Autodesk Fusion 360 part; units mm, degrees
(part 3 of 3)
sketch "Sketch8" plane through (0, 0, 8.15) normal (0, 0, 1) x (1, 0, 0) in component "Top"
extrude "Extrude4'" cut sketch "eaeb931b339a04fc4a439f0e48c97f53086cf32d_switch" along normal up to surface (1.5 mm away) contours L200 L201 L202 L203 bodies 1 in component "Plate"
sketch "Sketch9" plane through (0, 0, 8.15) normal (0, 0, 1) x (-1, 0, 0) in component "Top"
  line L0 (-81.77, -114.5353) -> (-67.7693, -114.5353)
  line L1 (-67.7693, -114.5353) -> (-67.7693, -128.5347)
  line L2 (-67.7693, -128.5347) -> (-81.77, -128.5347)
  line L3 (-81.77, -128.5347) -> (-81.77, -114.5353)
  circle A0 centre (-85.4771, -7.1284) radius 1
  circle A1 centre (-6.9121, -7.1284) radius 1
  circle A2 centre (-84.7093, -138.9743) radius 1
  line L4 (-81.77, -72.4598) -> (-81.77, -58.4606)
  line L5 (-81.77, -58.4606) -> (-77.0696, -58.4606)
  line L6 (-77.0696, -58.4606) -> (-77.0696, -56.9352)
  line L7 (-77.0696, -56.9352) -> (-80.2996, -56.9352)
  line L8 (-80.2996, -56.9352) -> (-80.2996, -55.2097)
  line L9 (-80.2996, -55.2097) -> (-81.219, -55.2097)
  line L10 (-81.219, -55.2097) -> (-81.219, -51.9105)
  line L11 (-81.219, -51.9105) -> (-80.2996, -51.9105)
  line L12 (-80.2996, -51.9105) -> (-80.2996, -50.1855)
  line L13 (-80.2996, -50.1855) -> (-77.0696, -50.1855)
  line L14 (-77.0696, -50.1855) -> (-77.0696, -49.36)
  line L15 (-77.0696, -49.36) -> (-74.2692, -49.36)
  line L16 (-74.2692, -49.36) -> (-74.2692, -50.1855)
  line L17 (-74.2692, -50.1855) -> (-67.9993, -50.1855)
  line L18 (-67.9993, -50.1855) -> (-67.9993, -51.9105)
  line L19 (-67.9993, -51.9105) -> (-67.0197, -51.9105)
  line L20 (-67.0197, -51.9105) -> (-67.0197, -55.2097)
  line L21 (-67.0197, -55.2097) -> (-67.9993, -55.2097)
  line L22 (-67.9993, -55.2097) -> (-67.9993, -56.9352)
  line L23 (-67.9993, -56.9352) -> (-72.4697, -56.9352)
  line L24 (-72.4697, -56.9352) -> (-72.4697, -58.4606)
  line L25 (-72.4697, -58.4606) -> (-67.7693, -58.4606)
  line L26 (-67.7693, -58.4606) -> (-67.7693, -72.4598)
  line L27 (-67.7693, -72.4598) -> (-72.4697, -72.4598)
  line L28 (-72.4697, -72.4598) -> (-72.4697, -73.9856)
  line L29 (-72.4697, -73.9856) -> (-67.9993, -73.9856)
  line L30 (-67.9993, -73.9856) -> (-67.9993, -75.7107)
  line L31 (-67.9993, -75.7107) -> (-67.0197, -75.7107)
  line L32 (-67.0197, -75.7107) -> (-67.0197, -79.0099)
  line L33 (-67.0197, -79.0099) -> (-67.9993, -79.0099)
  line L34 (-67.9993, -79.0099) -> (-67.9993, -80.735)
  line L35 (-67.9993, -80.735) -> (-74.2692, -80.735)
  line L36 (-74.2692, -80.735) -> (-74.2692, -81.5605)
  line L37 (-74.2692, -81.5605) -> (-77.0696, -81.5605)
  line L38 (-77.0696, -81.5605) -> (-77.0696, -80.735)
  line L39 (-77.0696, -80.735) -> (-80.2996, -80.735)
  line L40 (-80.2996, -80.735) -> (-80.2996, -79.0099)
  line L41 (-80.2996, -79.0099) -> (-81.219, -79.0099)
  line L42 (-81.219, -79.0099) -> (-81.219, -75.7107)
  line L43 (-81.219, -75.7107) -> (-80.2996, -75.7107)
  line L44 (-80.2996, -75.7107) -> (-80.2996, -73.9856)
  line L45 (-80.2996, -73.9856) -> (-77.0696, -73.9856)
  line L46 (-77.0696, -73.9856) -> (-77.0696, -72.4598)
  line L47 (-77.0696, -72.4598) -> (-81.77, -72.4598)
  line L48 (-24.62, -101.035) -> (-24.62, -87.0356)
  line L49 (-24.62, -87.0356) -> (-10.6192, -87.0356)
  line L50 (-10.6192, -87.0356) -> (-10.6192, -101.035)
  line L51 (-10.6192, -101.035) -> (-24.62, -101.035)
  line L52 (-31.4446, -129.035) -> (-60.9446, -129.035)
  line L53 (-60.9446, -129.035) -> (-60.9446, -114.035)
  line L54 (-60.9446, -114.035) -> (-31.4446, -114.035)
  line L55 (-31.4446, -114.035) -> (-31.4446, -129.035)
  line L56 (-10.6192, -114.5353) -> (-10.6192, -128.5347)
  line L57 (-10.6192, -128.5347) -> (-24.62, -128.5347)
  line L58 (-24.62, -128.5347) -> (-24.62, -114.5353)
  line L59 (-24.62, -114.5353) -> (-10.6192, -114.5353)
  line L60 (-24.62, -67.9856) -> (-10.6192, -67.9856)
  line L61 (-10.6192, -67.9856) -> (-10.6192, -81.9848)
  line L62 (-10.6192, -81.9848) -> (-24.62, -81.9848)
  line L63 (-24.62, -81.9848) -> (-24.62, -67.9856)
  line L64 (-48.7193, -101.035) -> (-62.72, -101.035)
  line L65 (-62.72, -101.035) -> (-62.72, -87.0356)
  line L66 (-62.72, -87.0356) -> (-48.7193, -87.0356)
  line L67 (-48.7193, -87.0356) -> (-48.7193, -101.035)
  line L68 (-81.77, -87.0356) -> (-67.7693, -87.0356)
  line L69 (-67.7693, -87.0356) -> (-67.7693, -101.035)
  line L70 (-67.7693, -101.035) -> (-81.77, -101.035)
  line L71 (-81.77, -101.035) -> (-81.77, -87.0356)
  line L72 (-62.72, -67.9856) -> (-48.7193, -67.9856)
  line L73 (-48.7193, -67.9856) -> (-48.7193, -81.9848)
  line L74 (-48.7193, -81.9848) -> (-62.72, -81.9848)
  line L75 (-62.72, -81.9848) -> (-62.72, -67.9856)
  line L76 (-29.6692, -67.9856) -> (-29.6692, -81.9848)
  line L77 (-29.6692, -81.9848) -> (-43.67, -81.9848)
  line L78 (-43.67, -81.9848) -> (-43.67, -67.9856)
  line L79 (-43.67, -67.9856) -> (-29.6692, -67.9856)
  line L80 (-29.6692, -48.9356) -> (-29.6692, -62.9348)
  line L81 (-29.6692, -62.9348) -> (-43.67, -62.9348)
  line L82 (-43.67, -62.9348) -> (-43.67, -48.9356)
  line L83 (-43.67, -48.9356) -> (-29.6692, -48.9356)
  line L84 (-67.9993, -12.0854) -> (-67.9993, -13.8107)
  line L85 (-67.9993, -13.8107) -> (-67.0197, -13.8107)
  line L86 (-67.0197, -13.8107) -> (-67.0197, -17.1097)
  line L87 (-67.0197, -17.1097) -> (-67.9993, -17.1097)
  line L88 (-67.9993, -17.1097) -> (-67.9993, -18.835)
  line L89 (-67.9993, -18.835) -> (-72.4697, -18.835)
  line L90 (-72.4697, -18.835) -> (-72.4697, -20.3605)
  line L91 (-72.4697, -20.3605) -> (-67.7693, -20.3605)
  line L92 (-67.7693, -20.3605) -> (-67.7693, -34.36)
  line L93 (-67.7693, -34.36) -> (-72.4697, -34.36)
  line L94 (-72.4697, -34.36) -> (-72.4697, -35.8856)
  line L95 (-72.4697, -35.8856) -> (-67.9993, -35.8856)
  line L96 (-67.9993, -35.8856) -> (-67.9993, -37.6107)
  line L97 (-67.9993, -37.6107) -> (-67.0197, -37.6107)
  line L98 (-67.0197, -37.6107) -> (-67.0197, -40.9099)
  line L99 (-67.0197, -40.9099) -> (-67.9993, -40.9099)
  line L100 (-67.9993, -40.9099) -> (-67.9993, -42.635)
  line L101 (-67.9993, -42.635) -> (-74.2692, -42.635)
  line L102 (-74.2692, -42.635) -> (-74.2692, -43.4605)
  line L103 (-74.2692, -43.4605) -> (-77.0696, -43.4605)
  line L104 (-77.0696, -43.4605) -> (-77.0696, -42.635)
  line L105 (-77.0696, -42.635) -> (-80.2996, -42.635)
  line L106 (-80.2996, -42.635) -> (-80.2996, -40.9099)
  line L107 (-80.2996, -40.9099) -> (-81.219, -40.9099)
  line L108 (-81.219, -40.9099) -> (-81.219, -37.6107)
  line L109 (-81.219, -37.6107) -> (-80.2996, -37.6107)
  line L110 (-80.2996, -37.6107) -> (-80.2996, -35.8856)
  line L111 (-80.2996, -35.8856) -> (-77.0696, -35.8856)
  line L112 (-77.0696, -35.8856) -> (-77.0696, -34.36)
  line L113 (-77.0696, -34.36) -> (-81.77, -34.36)
  line L114 (-81.77, -34.36) -> (-81.77, -20.3605)
  line L115 (-81.77, -20.3605) -> (-77.0696, -20.3605)
  line L116 (-77.0696, -20.3605) -> (-77.0696, -18.835)
  line L117 (-77.0696, -18.835) -> (-80.2996, -18.835)
  line L118 (-80.2996, -18.835) -> (-80.2996, -17.1097)
  line L119 (-80.2996, -17.1097) -> (-81.219, -17.1097)
  line L120 (-81.219, -17.1097) -> (-81.219, -13.8107)
  line L121 (-81.219, -13.8107) -> (-80.2996, -13.8107)
  line L122 (-80.2996, -13.8107) -> (-80.2996, -12.0854)
  line L123 (-80.2996, -12.0854) -> (-77.0696, -12.0854)
  line L124 (-77.0696, -12.0854) -> (-77.0696, -11.26)
  line L125 (-77.0696, -11.26) -> (-74.2692, -11.26)
  line L126 (-74.2692, -11.26) -> (-74.2692, -12.0854)
  line L127 (-74.2692, -12.0854) -> (-67.9993, -12.0854)
  line L128 (-48.7193, -62.9348) -> (-62.72, -62.9348)
  line L129 (-62.72, -62.9348) -> (-62.72, -48.9356)
  line L130 (-62.72, -48.9356) -> (-48.7193, -48.9356)
  line L131 (-48.7193, -48.9356) -> (-48.7193, -62.9348)
  line L132 (-48.7193, -10.8355) -> (-48.7193, -24.835)
  line L133 (-48.7193, -24.835) -> (-62.72, -24.835)
  line L134 (-62.72, -24.835) -> (-62.72, -10.8355)
  line L135 (-62.72, -10.8355) -> (-48.7193, -10.8355)
  line L136 (-37.3944, -23.3646) -> (-37.3944, -24.2852)
  line L137 (-37.3944, -24.2852) -> (-40.6936, -24.2852)
  line L138 (-40.6936, -24.2852) -> (-40.6936, -23.3646)
  line L139 (-40.6936, -23.3646) -> (-42.4187, -23.3646)
  line L140 (-42.4187, -23.3646) -> (-42.4187, -20.1345)
  line L141 (-42.4187, -20.1345) -> (-43.2442, -20.1345)
  line L142 (-43.2442, -20.1345) -> (-43.2442, -17.3357)
  line L143 (-43.2442, -17.3357) -> (-42.4187, -17.3357)
  line L144 (-42.4187, -17.3357) -> (-42.4187, -11.0657)
  line L145 (-42.4187, -11.0657) -> (-40.6936, -11.0657)
  line L146 (-40.6936, -11.0657) -> (-40.6936, -10.0858)
  line L147 (-40.6936, -10.0858) -> (-37.3944, -10.0858)
  line L148 (-37.3944, -10.0858) -> (-37.3944, -11.0657)
  line L149 (-37.3944, -11.0657) -> (-35.669, -11.0657)
  line L150 (-35.669, -11.0657) -> (-35.669, -15.5346)
  line L151 (-35.669, -15.5346) -> (-34.145, -15.5346)
  line L152 (-34.145, -15.5346) -> (-34.145, -10.8355)
  line L153 (-34.145, -10.8355) -> (-20.1442, -10.8355)
  line L154 (-20.1442, -10.8355) -> (-20.1442, -15.5346)
  line L155 (-20.1442, -15.5346) -> (-18.6201, -15.5346)
  line L156 (-18.6201, -15.5346) -> (-18.6201, -11.0657)
  line L157 (-18.6201, -11.0657) -> (-16.8934, -11.0657)
  line L158 (-16.8934, -11.0657) -> (-16.8934, -10.0858)
  line L159 (-16.8934, -10.0858) -> (-13.593, -10.0858)
  line L160 (-13.593, -10.0858) -> (-13.593, -11.0657)
  line L161 (-13.593, -11.0657) -> (-11.869, -11.0657)
  line L162 (-11.869, -11.0657) -> (-11.869, -17.3357)
  line L163 (-11.869, -17.3357) -> (-11.0436, -17.3357)
  line L164 (-11.0436, -17.3357) -> (-11.0436, -20.1345)
  line L165 (-11.0436, -20.1345) -> (-11.869, -20.1345)
  line L166 (-11.869, -20.1345) -> (-11.869, -23.3646)
  line L167 (-11.869, -23.3646) -> (-13.593, -23.3646)
  line L168 (-13.593, -23.3646) -> (-13.593, -24.2852)
  line L169 (-13.593, -24.2852) -> (-16.8934, -24.2852)
  line L170 (-16.8934, -24.2852) -> (-16.8934, -23.3646)
  line L171 (-16.8934, -23.3646) -> (-18.6201, -23.3646)
  line L172 (-18.6201, -23.3646) -> (-18.6201, -20.1345)
  line L173 (-18.6201, -20.1345) -> (-20.1442, -20.1345)
  line L174 (-20.1442, -20.1345) -> (-20.1442, -24.835)
  line L175 (-20.1442, -24.835) -> (-34.145, -24.835)
  line L176 (-34.145, -24.835) -> (-34.145, -20.1345)
  line L177 (-34.145, -20.1345) -> (-35.669, -20.1345)
  line L178 (-35.669, -20.1345) -> (-35.669, -23.3646)
  line L179 (-35.669, -23.3646) -> (-37.3944, -23.3646)
  line L180 (-62.72, -43.8849) -> (-62.72, -29.8855)
  line L181 (-62.72, -29.8855) -> (-48.7193, -29.8855)
  line L182 (-48.7193, -29.8855) -> (-48.7193, -43.8849)
  line L183 (-48.7193, -43.8849) -> (-62.72, -43.8849)
  line L184 (-24.62, -62.9348) -> (-24.62, -48.9356)
  line L185 (-24.62, -48.9356) -> (-10.6192, -48.9356)
  line L186 (-10.6192, -48.9356) -> (-10.6192, -62.9348)
  line L187 (-10.6192, -62.9348) -> (-24.62, -62.9348)
  line L188 (-43.67, -87.0356) -> (-29.6692, -87.0356)
  line L189 (-29.6692, -87.0356) -> (-29.6692, -101.035)
  line L190 (-29.6692, -101.035) -> (-43.67, -101.035)
  line L191 (-43.67, -101.035) -> (-43.67, -87.0356)
  line L192 (-24.62, -43.8849) -> (-24.62, -29.8855)
  line L193 (-24.62, -29.8855) -> (-10.6192, -29.8855)
  line L194 (-10.6192, -29.8855) -> (-10.6192, -43.8849)
  line L195 (-10.6192, -43.8849) -> (-24.62, -43.8849)
  line L196 (-29.6692, -29.8855) -> (-29.6692, -43.8849)
  line L197 (-29.6692, -43.8849) -> (-43.67, -43.8849)
  line L198 (-43.67, -43.8849) -> (-43.67, -29.8855)
  line L199 (-43.67, -29.8855) -> (-29.6692, -29.8855)
  arc A3 (-6.6192, -142.035) -> (-4.6192, -140.035) centre (-6.6192, -140.035) ccw
  line L200 (-4.6192, -140.035) -> (-4.6192, -6.8355)
  arc A4 (-4.6192, -6.8355) -> (-6.6192, -4.8355) centre (-6.6192, -6.8355) ccw
  line L201 (-6.6192, -4.8355) -> (-85.77, -4.8355)
  arc A5 (-85.77, -4.8355) -> (-87.77, -6.8355) centre (-85.77, -6.8355) ccw
  line L202 (-87.77, -6.8355) -> (-87.77, -140.035)
  arc A6 (-87.77, -140.035) -> (-85.77, -142.035) centre (-85.77, -140.035) ccw
  line L203 (-85.77, -142.035) -> (-6.6192, -142.035)
extrude "Extrude11" cut sketch "Sketch9" against normal up to surface (6.65 mm away) contours L52 L53 L54 L55 bodies 2 in component "Top"
fillet "Fillet6" radius 1 4 edges at (60.9446, 129.035, 4.9) (31.4446, 129.035, 4.9) (31.4446, 114.035, 4.9) (60.9446, 114.035, 4.9) on bodies 2 in component "Top"
extrude "Extrude10" [suppressed] in component "Top"
ref_plane "WorkPlane3" through (46.1946, 67.8413, 1.075) normal (0, 0, -1) x (-1, 0, 0) in component "Top"
sketch "Sketch2 (2)" plane through (0, 0, -13) normal (0, 0, -1) x (1, 0, 0) in component "Bottom"
  arc A0 (-1.5308, 3.3145) -> (-3.5308, 1.3145) centre (-1.5308, 1.3145) ccw
  line L0 (-3.5308, 1.3145) -> (-3.5308, -136.997)
  arc A1 (-3.5308, -136.997) -> (-1.5308, -138.997) centre (-1.5308, -136.997) ccw
  line L1 (-1.5308, -138.997) -> (93.92, -138.997)
  arc A2 (93.92, -138.997) -> (95.92, -136.997) centre (93.92, -136.997) ccw
  line L2 (95.92, -136.997) -> (95.92, 1.3145)
  arc A3 (95.92, 1.3145) -> (93.92, 3.3145) centre (93.92, 1.3145) ccw
  line L3 (93.92, 3.3145) -> (-1.5308, 3.3145)
  line L4 (-3.5308, -138.997) -> (0.4692, -138.997) construction
  line L5 (0.4692, -138.997) -> (0.4692, -134.997) construction
  line L6 (0.4692, -134.997) -> (-3.5308, -134.997) construction
  line L7 (-3.5308, -138.997) -> (-3.5308, -134.997) construction
  circle A4 centre (0.4692, -134.997) radius 1.5
  dimension "d137" = 4
  dimension "d138" = 4
  dimension "d139" = 3
  constraint perpendicular L0 L4
  constraint perpendicular L4 L5
  constraint coincident L0 L6.end
  constraint perpendicular L0 L6
  constraint perpendicular L6 L7
  constraint coincident L5.end L6.start
  measures "d137" distance of L4.start L4.end
  measures "d138" distance of L4.end L5.end
  measures "d139" diameter of A4
extrude "Extrude8" [suppressed] in component "Top"
extrude "Extrude2''" [no effect] in component "Lit Stripe"
extrude "Extrude2'''" [no effect] in component "Bottom"
mirror "Mirror3" [suppressed] in component "Top"
mirror "Mirror1''" [no effect] in component "Lit Stripe"
mirror "Mirror1'''" [no effect] in component "Bottom"
mirror "Mirror4" [suppressed] in component "Top"
mirror "Mirror2''" [no effect] in component "Lit Stripe"
mirror "Mirror2'''" [no effect] in component "Bottom"
sketch "Sketch3 (3)" plane through (0, 0, -13) normal (0, 0, -1) x (1, 0, 0) in component "Bottom"
  circle A0 centre (91.92, -0.6855) radius 1.5
  circle A1 centre (0.4692, -0.6855) radius 1.5
  circle A2 centre (91.92, -134.997) radius 1.5
  circle A3 centre (0.4692, -134.997) radius 1.5
  arc A4 (-1.5308, 3.3145) -> (-3.5308, 1.3145) centre (-1.5308, 1.3145) ccw
  line L0 (-3.5308, 1.3145) -> (-3.5308, -136.997)
  arc A5 (-3.5308, -136.997) -> (-1.5308, -138.997) centre (-1.5308, -136.997) ccw
  line L1 (-1.5308, -138.997) -> (93.92, -138.997)
  arc A6 (93.92, -138.997) -> (95.92, -136.997) centre (93.92, -136.997) ccw
  line L2 (95.92, -136.997) -> (95.92, 1.3145)
  arc A7 (95.92, 1.3145) -> (93.92, 3.3145) centre (93.92, 1.3145) ccw
  line L3 (93.92, 3.3145) -> (-1.5308, 3.3145)
  line L4 (91.92, -0.6855) -> (91.92, -134.997) construction
  line L5 (95.92, -67.8413) -> (-3.5308, -67.8412) construction
  circle A8 centre (91.92, -67.8413) radius 1.5
  dimension "d152" = 3
  constraint coincident A0.centre L4.start
  constraint coincident A2.centre L4.end
  constraint midpoint L2 L5.start
  constraint midpoint L0 L5.end
  constraint midpoint L4 A8.centre
  measures "d152" diameter of A8
extrude "Extrude9" [suppressed] in component "Top"
extrude "Extrude3''" [no effect] in component "Lit Stripe"
extrude "Extrude3'''" [no effect] in component "Bottom"
mirror "Mirror5" [suppressed] in component "Top"
mirror "Mirror3'" [no effect] in component "Lit Stripe"
mirror "Mirror3''" [no effect] in component "Bottom"
sketch "Sketch4 (2)" plane through (0, 0, 1.5) normal (0, 0, 1) x (-1, 0, 0) in component "Top"
  circle A0 centre (-85.4771, -7.1284) radius 1
  circle A1 centre (-6.9121, -7.1284) radius 1
  circle A2 centre (-84.4771, -127.5541) radius 1
  circle A3 centre (-7.9121, -127.5541) radius 1
  line L0 (-34.1946, -124.3473) -> (-58.1946, -124.3473)
  line L1 (-58.1946, -124.3473) -> (-58.1946, -111.3473)
  line L2 (-58.1946, -111.3473) -> (-34.1946, -111.3473)
  line L3 (-34.1946, -111.3473) -> (-34.1946, -124.3473)
  line L4 (-81.77, -72.4598) -> (-81.77, -58.4606)
  line L5 (-81.77, -58.4606) -> (-77.0696, -58.4606)
  line L6 (-77.0696, -58.4606) -> (-77.0696, -56.9352)
  line L7 (-77.0696, -56.9352) -> (-80.2996, -56.9352)
  line L8 (-80.2996, -56.9352) -> (-80.2996, -55.2097)
  line L9 (-80.2996, -55.2097) -> (-81.219, -55.2097)
  line L10 (-81.219, -55.2097) -> (-81.219, -51.9105)
  line L11 (-81.219, -51.9105) -> (-80.2996, -51.9105)
  line L12 (-80.2996, -51.9105) -> (-80.2996, -50.1855)
  line L13 (-80.2996, -50.1855) -> (-77.0696, -50.1855)
  line L14 (-77.0696, -50.1855) -> (-77.0696, -49.36)
  line L15 (-77.0696, -49.36) -> (-74.2692, -49.36)
  line L16 (-74.2692, -49.36) -> (-74.2692, -50.1855)
  line L17 (-74.2692, -50.1855) -> (-67.9993, -50.1855)
  line L18 (-67.9993, -50.1855) -> (-67.9993, -51.9105)
  line L19 (-67.9993, -51.9105) -> (-67.0197, -51.9105)
  line L20 (-67.0197, -51.9105) -> (-67.0197, -55.2097)
  line L21 (-67.0197, -55.2097) -> (-67.9993, -55.2097)
  line L22 (-67.9993, -55.2097) -> (-67.9993, -56.9352)
  line L23 (-67.9993, -56.9352) -> (-72.4697, -56.9352)
  line L24 (-72.4697, -56.9352) -> (-72.4697, -58.4606)
  line L25 (-72.4697, -58.4606) -> (-67.7693, -58.4606)
  line L26 (-67.7693, -58.4606) -> (-67.7693, -72.4598)
  line L27 (-67.7693, -72.4598) -> (-72.4697, -72.4598)
  line L28 (-72.4697, -72.4598) -> (-72.4697, -73.9856)
  line L29 (-72.4697, -73.9856) -> (-67.9993, -73.9856)
  line L30 (-67.9993, -73.9856) -> (-67.9993, -75.7107)
  line L31 (-67.9993, -75.7107) -> (-67.0197, -75.7107)
  line L32 (-67.0197, -75.7107) -> (-67.0197, -79.0099)
  line L33 (-67.0197, -79.0099) -> (-67.9993, -79.0099)
  line L34 (-67.9993, -79.0099) -> (-67.9993, -80.735)
  line L35 (-67.9993, -80.735) -> (-74.2692, -80.735)
  line L36 (-74.2692, -80.735) -> (-74.2692, -81.5605)
  line L37 (-74.2692, -81.5605) -> (-77.0696, -81.5605)
  line L38 (-77.0696, -81.5605) -> (-77.0696, -80.735)
  line L39 (-77.0696, -80.735) -> (-80.2996, -80.735)
  line L40 (-80.2996, -80.735) -> (-80.2996, -79.0099)
  line L41 (-80.2996, -79.0099) -> (-81.219, -79.0099)
  line L42 (-81.219, -79.0099) -> (-81.219, -75.7107)
  line L43 (-81.219, -75.7107) -> (-80.2996, -75.7107)
  line L44 (-80.2996, -75.7107) -> (-80.2996, -73.9856)
  line L45 (-80.2996, -73.9856) -> (-77.0696, -73.9856)
  line L46 (-77.0696, -73.9856) -> (-77.0696, -72.4598)
  line L47 (-77.0696, -72.4598) -> (-81.77, -72.4598)
  line L48 (-24.62, -67.9856) -> (-10.6192, -67.9856)
  line L49 (-10.6192, -67.9856) -> (-10.6192, -81.9848)
  line L50 (-10.6192, -81.9848) -> (-24.62, -81.9848)
  line L51 (-24.62, -81.9848) -> (-24.62, -67.9856)
  line L52 (-10.6192, -110.8476) -> (-10.6192, -124.847)
  line L53 (-10.6192, -124.847) -> (-24.62, -124.847)
  line L54 (-24.62, -124.847) -> (-24.62, -110.8476)
  line L55 (-24.62, -110.8476) -> (-10.6192, -110.8476)
  line L56 (-24.62, -101.035) -> (-24.62, -87.0356)
  line L57 (-24.62, -87.0356) -> (-10.6192, -87.0356)
  line L58 (-10.6192, -87.0356) -> (-10.6192, -101.035)
  line L59 (-10.6192, -101.035) -> (-24.62, -101.035)
  line L60 (-29.6692, -48.9356) -> (-29.6692, -62.9348)
  line L61 (-29.6692, -62.9348) -> (-43.67, -62.9348)
  line L62 (-43.67, -62.9348) -> (-43.67, -48.9356)
  line L63 (-43.67, -48.9356) -> (-29.6692, -48.9356)
  line L64 (-29.6692, -67.9856) -> (-29.6692, -81.9848)
  line L65 (-29.6692, -81.9848) -> (-43.67, -81.9848)
  line L66 (-43.67, -81.9848) -> (-43.67, -67.9856)
  line L67 (-43.67, -67.9856) -> (-29.6692, -67.9856)
  line L68 (-62.72, -67.9856) -> (-48.7193, -67.9856)
  line L69 (-48.7193, -67.9856) -> (-48.7193, -81.9848)
  line L70 (-48.7193, -81.9848) -> (-62.72, -81.9848)
  line L71 (-62.72, -81.9848) -> (-62.72, -67.9856)
  line L72 (-81.77, -87.0356) -> (-67.7693, -87.0356)
  line L73 (-67.7693, -87.0356) -> (-67.7693, -101.035)
  line L74 (-67.7693, -101.035) -> (-81.77, -101.035)
  line L75 (-81.77, -101.035) -> (-81.77, -87.0356)
  line L76 (-48.7193, -101.035) -> (-62.72, -101.035)
  line L77 (-62.72, -101.035) -> (-62.72, -87.0356)
  line L78 (-62.72, -87.0356) -> (-48.7193, -87.0356)
  line L79 (-48.7193, -87.0356) -> (-48.7193, -101.035)
  line L80 (-67.9993, -12.0854) -> (-67.9993, -13.8107)
  line L81 (-67.9993, -13.8107) -> (-67.0197, -13.8107)
  line L82 (-67.0197, -13.8107) -> (-67.0197, -17.1097)
  line L83 (-67.0197, -17.1097) -> (-67.9993, -17.1097)
  line L84 (-67.9993, -17.1097) -> (-67.9993, -18.835)
  line L85 (-67.9993, -18.835) -> (-72.4697, -18.835)
  line L86 (-72.4697, -18.835) -> (-72.4697, -20.3605)
  line L87 (-72.4697, -20.3605) -> (-67.7693, -20.3605)
  line L88 (-67.7693, -20.3605) -> (-67.7693, -34.36)
  line L89 (-67.7693, -34.36) -> (-72.4697, -34.36)
  line L90 (-72.4697, -34.36) -> (-72.4697, -35.8856)
  line L91 (-72.4697, -35.8856) -> (-67.9993, -35.8856)
  line L92 (-67.9993, -35.8856) -> (-67.9993, -37.6107)
  line L93 (-67.9993, -37.6107) -> (-67.0197, -37.6107)
  line L94 (-67.0197, -37.6107) -> (-67.0197, -40.9099)
  line L95 (-67.0197, -40.9099) -> (-67.9993, -40.9099)
  line L96 (-67.9993, -40.9099) -> (-67.9993, -42.635)
  line L97 (-67.9993, -42.635) -> (-74.2692, -42.635)
  line L98 (-74.2692, -42.635) -> (-74.2692, -43.4605)
  line L99 (-74.2692, -43.4605) -> (-77.0696, -43.4605)
  line L100 (-77.0696, -43.4605) -> (-77.0696, -42.635)
  line L101 (-77.0696, -42.635) -> (-80.2996, -42.635)
  line L102 (-80.2996, -42.635) -> (-80.2996, -40.9099)
  line L103 (-80.2996, -40.9099) -> (-81.219, -40.9099)
  line L104 (-81.219, -40.9099) -> (-81.219, -37.6107)
  line L105 (-81.219, -37.6107) -> (-80.2996, -37.6107)
  line L106 (-80.2996, -37.6107) -> (-80.2996, -35.8856)
  line L107 (-80.2996, -35.8856) -> (-77.0696, -35.8856)
  line L108 (-77.0696, -35.8856) -> (-77.0696, -34.36)
  line L109 (-77.0696, -34.36) -> (-81.77, -34.36)
  line L110 (-81.77, -34.36) -> (-81.77, -20.3605)
  line L111 (-81.77, -20.3605) -> (-77.0696, -20.3605)
  line L112 (-77.0696, -20.3605) -> (-77.0696, -18.835)
  line L113 (-77.0696, -18.835) -> (-80.2996, -18.835)
  line L114 (-80.2996, -18.835) -> (-80.2996, -17.1097)
  line L115 (-80.2996, -17.1097) -> (-81.219, -17.1097)
  line L116 (-81.219, -17.1097) -> (-81.219, -13.8107)
  line L117 (-81.219, -13.8107) -> (-80.2996, -13.8107)
  line L118 (-80.2996, -13.8107) -> (-80.2996, -12.0854)
  line L119 (-80.2996, -12.0854) -> (-77.0696, -12.0854)
  line L120 (-77.0696, -12.0854) -> (-77.0696, -11.26)
  line L121 (-77.0696, -11.26) -> (-74.2692, -11.26)
  line L122 (-74.2692, -11.26) -> (-74.2692, -12.0854)
  line L123 (-74.2692, -12.0854) -> (-67.9993, -12.0854)
  line L124 (-48.7193, -62.9348) -> (-62.72, -62.9348)
  line L125 (-62.72, -62.9348) -> (-62.72, -48.9356)
  line L126 (-62.72, -48.9356) -> (-48.7193, -48.9356)
  line L127 (-48.7193, -48.9356) -> (-48.7193, -62.9348)
  line L128 (-48.7193, -10.8355) -> (-48.7193, -24.835)
  line L129 (-48.7193, -24.835) -> (-62.72, -24.835)
  line L130 (-62.72, -24.835) -> (-62.72, -10.8355)
  line L131 (-62.72, -10.8355) -> (-48.7193, -10.8355)
  line L132 (-37.3944, -23.3646) -> (-37.3944, -24.2852)
  line L133 (-37.3944, -24.2852) -> (-40.6936, -24.2852)
  line L134 (-40.6936, -24.2852) -> (-40.6936, -23.3646)
  line L135 (-40.6936, -23.3646) -> (-42.4187, -23.3646)
  line L136 (-42.4187, -23.3646) -> (-42.4187, -20.1345)
  line L137 (-42.4187, -20.1345) -> (-43.2442, -20.1345)
  line L138 (-43.2442, -20.1345) -> (-43.2442, -17.3357)
  line L139 (-43.2442, -17.3357) -> (-42.4187, -17.3357)
  line L140 (-42.4187, -17.3357) -> (-42.4187, -11.0657)
  line L141 (-42.4187, -11.0657) -> (-40.6936, -11.0657)
  line L142 (-40.6936, -11.0657) -> (-40.6936, -10.0858)
  line L143 (-40.6936, -10.0858) -> (-37.3944, -10.0858)
  line L144 (-37.3944, -10.0858) -> (-37.3944, -11.0657)
  line L145 (-37.3944, -11.0657) -> (-35.669, -11.0657)
  line L146 (-35.669, -11.0657) -> (-35.669, -15.5346)
  line L147 (-35.669, -15.5346) -> (-34.145, -15.5346)
  line L148 (-34.145, -15.5346) -> (-34.145, -10.8355)
  line L149 (-34.145, -10.8355) -> (-20.1442, -10.8355)
  line L150 (-20.1442, -10.8355) -> (-20.1442, -15.5346)
  line L151 (-20.1442, -15.5346) -> (-18.6201, -15.5346)
  line L152 (-18.6201, -15.5346) -> (-18.6201, -11.0657)
  line L153 (-18.6201, -11.0657) -> (-16.8934, -11.0657)
  line L154 (-16.8934, -11.0657) -> (-16.8934, -10.0858)
  line L155 (-16.8934, -10.0858) -> (-13.593, -10.0858)
  line L156 (-13.593, -10.0858) -> (-13.593, -11.0657)
  line L157 (-13.593, -11.0657) -> (-11.869, -11.0657)
  line L158 (-11.869, -11.0657) -> (-11.869, -17.3357)
  line L159 (-11.869, -17.3357) -> (-11.0436, -17.3357)
  line L160 (-11.0436, -17.3357) -> (-11.0436, -20.1345)
  line L161 (-11.0436, -20.1345) -> (-11.869, -20.1345)
  line L162 (-11.869, -20.1345) -> (-11.869, -23.3646)
  line L163 (-11.869, -23.3646) -> (-13.593, -23.3646)
  line L164 (-13.593, -23.3646) -> (-13.593, -24.2852)
  line L165 (-13.593, -24.2852) -> (-16.8934, -24.2852)
  line L166 (-16.8934, -24.2852) -> (-16.8934, -23.3646)
  line L167 (-16.8934, -23.3646) -> (-18.6201, -23.3646)
  line L168 (-18.6201, -23.3646) -> (-18.6201, -20.1345)
  line L169 (-18.6201, -20.1345) -> (-20.1442, -20.1345)
  line L170 (-20.1442, -20.1345) -> (-20.1442, -24.835)
  line L171 (-20.1442, -24.835) -> (-34.145, -24.835)
  line L172 (-34.145, -24.835) -> (-34.145, -20.1345)
  line L173 (-34.145, -20.1345) -> (-35.669, -20.1345)
  line L174 (-35.669, -20.1345) -> (-35.669, -23.3646)
  line L175 (-35.669, -23.3646) -> (-37.3944, -23.3646)
  line L176 (-62.72, -43.8849) -> (-62.72, -29.8855)
  line L177 (-62.72, -29.8855) -> (-48.7193, -29.8855)
  line L178 (-48.7193, -29.8855) -> (-48.7193, -43.8849)
  line L179 (-48.7193, -43.8849) -> (-62.72, -43.8849)
  line L180 (-24.62, -62.9348) -> (-24.62, -48.9356)
  line L181 (-24.62, -48.9356) -> (-10.6192, -48.9356)
  line L182 (-10.6192, -48.9356) -> (-10.6192, -62.9348)
  line L183 (-10.6192, -62.9348) -> (-24.62, -62.9348)
  line L184 (-43.67, -87.0356) -> (-29.6692, -87.0356)
  line L185 (-29.6692, -87.0356) -> (-29.6692, -101.035)
  line L186 (-29.6692, -101.035) -> (-43.67, -101.035)
  line L187 (-43.67, -101.035) -> (-43.67, -87.0356)
  line L188 (-24.62, -43.8849) -> (-24.62, -29.8855)
  line L189 (-24.62, -29.8855) -> (-10.6192, -29.8855)
  line L190 (-10.6192, -29.8855) -> (-10.6192, -43.8849)
  line L191 (-10.6192, -43.8849) -> (-24.62, -43.8849)
  line L192 (-29.6692, -29.8855) -> (-29.6692, -43.8849)
  line L193 (-29.6692, -43.8849) -> (-43.67, -43.8849)
  line L194 (-43.67, -43.8849) -> (-43.67, -29.8855)
  line L195 (-43.67, -29.8855) -> (-29.6692, -29.8855)
  arc A4 (-6.6192, -130.847) -> (-4.6192, -128.847) centre (-6.6192, -128.847) ccw
  line L196 (-4.6192, -128.847) -> (-4.6192, -6.8355)
  arc A5 (-4.6192, -6.8355) -> (-6.6192, -4.8355) centre (-6.6192, -6.8355) ccw
  line L197 (-6.6192, -4.8355) -> (-85.77, -4.8355)
  arc A6 (-85.77, -4.8355) -> (-87.77, -6.8355) centre (-85.77, -6.8355) ccw
  line L198 (-87.77, -6.8355) -> (-87.77, -128.847)
  arc A7 (-87.77, -128.847) -> (-85.77, -130.847) centre (-85.77, -128.847) ccw
  line L199 (-85.77, -130.847) -> (-6.6192, -130.847)
  line L200 (-10.6192, -110.8476) -> (-10.6192, -124.847)
  line L201 (-24.62, -124.847) -> (-24.62, -110.8476)
  line L202 (-10.6192, -110.8476) -> (-24.62, -110.8476)
  line L203 (-24.62, -124.847) -> (-10.6192, -124.847)
  line L204 (-8.0892, -108.3176) -> (-8.0892, -127.377)
  line L205 (-27.15, -127.377) -> (-8.0892, -127.377)
  line L206 (-27.15, -127.377) -> (-27.15, -108.3176)
  line L207 (-8.0892, -108.3176) -> (-27.15, -108.3176)
  dimension "d166" = 2.53
  constraint coincident L52.start L55.end
  constraint coincident L52.end L53.start
  constraint coincident L53.end L54.start
  constraint coincident L54.end L55.start
component "Plate" placed x (1, 0, 0) y (0, 1, 0) z (0, 0, 1) at (0, 0, 0)
component "Top" placed x (1, 0, 0) y (0, 1, 0) z (0, 0, 1) at (0, 0, 0)
component "Lit Stripe" placed x (1, 0, 0) y (0, 1, 0) z (0, 0, 1) at (0, 0, 0)
component "Bottom" placed x (1, 0, 0) y (0, 1, 0) z (0, 0, 1) at (0, 0, 0)
